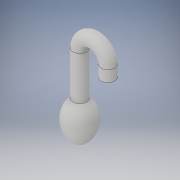
# Autodesk Inventor part: tail
Saved by Autodesk Inventor 2019.3 (Build 233278000, 278)
## iProperties
Created: 2019-02-15
Part Number: tail
Material: Generic
Document SubType Name: Modeling
Designer: Frienddo
Density: 1 g/cm^3
Appearance: Default
Author: Frienddo
Autodesk Inventor part; units mm, degrees
ref_plane "YZ Plane" through (0, 0, 0) normal (1, 0, 0) x (0, 1, 0)
ref_plane "XZ Plane" through (0, 0, 0) normal (0, 1, 0) x (-1, 0, 0)
ref_plane "XY Plane" through (0, 0, 0) normal (0, 0, 1) x (1, 0, 0)
sketch "Sketch1" plane through (0, 0, 0) normal (0, 1, 0) x (-1, 0, 0)
  circle A0 centre (0, 0) radius 3.2534
  constraints: 1 centre point, 1 coincident
sketch "Sketch2" plane through (0, 0, 0) normal (0, 0, 1) x (1, 0, 0)
  line L0 (0, 0) -> (0, 5.311)
  arc A0 (0, 5.311) -> (-13.4126, 5.311) centre (-6.7063, 5.311) ccw
  line L1 (-13.4126, 5.311) -> (-13.4126, -19.5678)
  constraints: 4 end point, 2 point on circle, 2 tangent, 1 centre point, 1 parallel, 1 vertical
sweep "Sweep1" add profiles "Sketch1" path "Sketch2"
sketch "Sketch3" plane through (0, 0, 0) normal (0, 0, 1) x (1, 0, 0)
  line L0 (-16.6659, -19.5678) -> (-10.1592, -19.5678) projected
  line L1 (-13.4126, -19.5678) -> (-13.4126, -13.216)
  line L2 (-13.4126, -34.4855) -> (-13.4126, -19.5678)
  line L3 (-13.4126, -13.216) -> (-13.4126, -12.2227)
  arc A0 (-13.4126, -13.216) -> (-13.4126, -34.4855) centre (-8.7099, -23.8508) ccw
  point P0 (0, 0)
  constraints: 6 end point, 3 vertical, 2 point on circle, 1 centre point, 1 midpoint
revolve "Revolution1" add sketch "Sketch3" angle 360 about axis through (-13.4126, -34.4855, 0) along (0, 1, 0)
body "Solid1"
